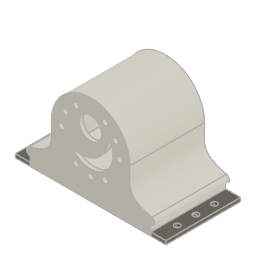
inspection_robot_01 (Autodesk Fusion 360 archive; units mm, degrees)
design "Motor Holder - JGB37-520"
Autodesk Fusion 360 part; units mm, degrees
sketch "Sketch1" plane through (0, 0, 0) normal (0, 1, 0) x (1, 0, 0)
  spline S0 degree 3 poles (32.2186, -5) (32.4791, -5) (32.737, -5.0509) (33.2189, -5.2486) (33.4382, -5.3936) (33.8089, -5.7595) (33.9568, -5.9769) (34.1608, -6.4561) (34.2151, -6.7133) (34.2219, -7.2342) (34.1744, -7.4927) (33.983, -7.9772) (33.8409, -8.1984) (33.5297, -8.5221) (33.3803, -8.6389) (33.0533, -8.8273) (32.8773, -8.8978) (32.6941, -8.9427) knots 0 0 0 0 0.078129 0.078129 0.156258 0.156258 0.234387 0.234387 0.312516 0.312516 0.390644 0.390644 0.468773 0.468773 0.525375 0.525375 0.581976 0.581976 0.581976 0.581976
  spline S1 degree 3 poles (32.6941, -8.9427) (29.0069, -9.845) (26.7125, -10.8301) (23.8662, -12.5388) (23.0225, -13.3268) (21.8903, -14.8113) (21.5152, -15.5908) (20.97, -17.528) (20.8705, -18.6908) (20.8263, -21.8742) (20.9873, -23.9601) (20.9873, -27) knots 0 0 0 0 1.138808 1.138808 2.091056 2.091056 2.992987 2.992987 4.085417 4.085417 5.724443 5.724443 5.724443 5.724443
  circle A0 centre (-0.0127, -34) radius 6
  spline S2 degree 3 poles (-32.7195, -8.9427) (-32.9724, -8.8808) (-33.2109, -8.77) (-33.6319, -8.4634) (-33.8105, -8.2705) (-34.0836, -7.8269) (-34.1756, -7.5806) (-34.2598, -7.0666) (-34.2514, -6.8039) (-34.1342, -6.2964) (-34.0266, -6.0565) (-33.7256, -5.6314) (-33.535, -5.4504) (-33.1557, -5.2099) (-32.9828, -5.1319) (-32.6205, -5.0267) (-32.4327, -5) (-32.2441, -5) knots 0 0 0 0 0.078129 0.078129 0.156258 0.156258 0.234387 0.234387 0.312516 0.312516 0.390644 0.390644 0.468773 0.468773 0.525375 0.525375 0.581976 0.581976 0.581976 0.581976
  circle A1 centre (7.7373, -13.5766) radius 1.5
  line L0 (32.2186, -5) -> (32.2186, 0)
  circle A2 centre (7.7373, -40.4234) radius 1.5
  arc A3 (9.7096, -34.034) -> (-9.7039, -19.9233) centre (-0.0127, -27) ccw
  arc A4 (-21.0127, -27) -> (20.9873, -27) centre (-0.0127, -27) ccw
  circle A5 centre (-0.0127, -11.5) radius 1.5
  spline S3 degree 3 poles (-21.0127, -27) (-21.0127, -21.6083) (-20.4943, -18.5071) (-21.8096, -15.0156) (-22.2712, -14.2366) (-23.6233, -12.8057) (-24.5151, -12.1033) (-27.7492, -10.3649) (-30.1557, -9.5701) (-32.7195, -8.9427) knots 0 0 0 0 1.617502 1.617502 2.113141 2.113141 2.569404 2.569404 3.248781 3.248781 3.248781 3.248781
  line L1 (-32.2441, 0) -> (-32.2441, -5)
  circle A6 centre (-13.4361, -34.75) radius 1.5
  circle A7 centre (-7.7627, -40.4234) radius 1.5
  circle A8 centre (13.4107, -34.75) radius 1.5
  circle A9 centre (-15.5127, -27) radius 1.5
  circle A10 centre (15.4873, -27) radius 1.5
  circle A11 centre (-7.7627, -13.5766) radius 1.5
  arc A12 (9.7096, -34.034) -> (-9.7039, -19.9233) centre (-5.2887, -34.2587) ccw
  line L2 (32.2186, 0) -> (-32.2441, 0)
  point P0 (-67.8, -16)
  constraint perpendicular L1 L2
extrude "Extrude1" add sketch "Sketch1" along normal blind 40 makes body 1
sketch "Sketch2" plane through (0, 40, 0) normal (0, 1, 0) x (-1, 0, 0)
  circle A0 centre (13.4361, 34.75) radius 1.5
  circle A1 centre (0.0127, 11.5) radius 1.5
  circle A2 centre (-15.4873, 27) radius 1.5
  circle A3 centre (-7.7373, 40.4234) radius 1.5
  circle A4 centre (7.7627, 40.4234) radius 1.5
  circle A5 centre (-13.4107, 34.75) radius 1.5
  circle A6 centre (7.7627, 13.5766) radius 1.5
  arc A7 (-9.7096, 34.034) -> (9.7039, 19.9233) centre (0.0127, 27) ccw
  arc A8 (-9.7096, 34.034) -> (9.7039, 19.9233) centre (5.2887, 34.2587) ccw
  circle A9 centre (15.5127, 27) radius 1.5
  line L0 (-32.2186, 5) -> (-32.2186, 0)
  line L1 (-32.2186, 0) -> (32.2441, 0)
  line L2 (32.2441, 0) -> (32.2441, 5)
  spline S0 degree 3 poles (32.2441, 5) (32.4327, 5) (32.6205, 5.0267) (32.9828, 5.1319) (33.1557, 5.2099) (33.535, 5.4504) (33.7256, 5.6314) (34.0266, 6.0565) (34.1342, 6.2964) (34.2514, 6.8039) (34.2598, 7.0666) (34.1756, 7.5806) (34.0836, 7.8269) (33.8105, 8.2705) (33.6319, 8.4634) (33.2109, 8.77) (32.9724, 8.8808) (32.7195, 8.9427) knots -0.581976 -0.581976 -0.581976 -0.581976 -0.525375 -0.525375 -0.468773 -0.468773 -0.390644 -0.390644 -0.312516 -0.312516 -0.234387 -0.234387 -0.156258 -0.156258 -0.078129 -0.078129 0 0 0 0
  spline S1 degree 3 poles (32.7195, 8.9427) (30.1557, 9.5701) (27.7492, 10.3649) (24.5151, 12.1033) (23.6233, 12.8057) (22.2712, 14.2366) (21.8096, 15.0156) (20.4943, 18.5071) (21.0127, 21.6083) (21.0127, 27) knots -3.248781 -3.248781 -3.248781 -3.248781 -2.569404 -2.569404 -2.113141 -2.113141 -1.617502 -1.617502 0 0 0 0
  arc A10 (21.0127, 27) -> (-20.9873, 27) centre (0.0127, 27) ccw
  spline S2 degree 3 poles (-20.9873, 27) (-20.9873, 23.9601) (-20.8263, 21.8742) (-20.8705, 18.6908) (-20.97, 17.528) (-21.5152, 15.5908) (-21.8903, 14.8113) (-23.0225, 13.3268) (-23.8662, 12.5388) (-26.7125, 10.8301) (-29.0069, 9.845) (-32.6941, 8.9427) knots -5.724443 -5.724443 -5.724443 -5.724443 -4.085417 -4.085417 -2.992987 -2.992987 -2.091056 -2.091056 -1.138808 -1.138808 0 0 0 0
  spline S3 degree 3 poles (-32.6941, 8.9427) (-32.8773, 8.8978) (-33.0533, 8.8273) (-33.3803, 8.6389) (-33.5297, 8.5221) (-33.8409, 8.1984) (-33.983, 7.9772) (-34.1744, 7.4927) (-34.2219, 7.2342) (-34.2151, 6.7133) (-34.1608, 6.4561) (-33.9568, 5.9769) (-33.8089, 5.7595) (-33.4382, 5.3936) (-33.2189, 5.2486) (-32.737, 5.0509) (-32.4791, 5) (-32.2186, 5) knots -0.581976 -0.581976 -0.581976 -0.581976 -0.525375 -0.525375 -0.468773 -0.468773 -0.390644 -0.390644 -0.312516 -0.312516 -0.234387 -0.234387 -0.156258 -0.156258 -0.078129 -0.078129 0 0 0 0
  circle A11 centre (-7.7373, 13.5766) radius 1.5
  circle A12 centre (0.0127, 34) radius 6
  arc A13 (-30.2186, 5) -> (-32.2186, 7) centre (-32.2186, 5) ccw
  line L3 (-30.2186, 5) -> (-30.2186, 2)
  line L4 (-30.2186, 2) -> (30.2441, 2)
  line L5 (30.2441, 2) -> (30.2441, 5)
  arc A14 (32.2441, 7) -> (30.2441, 5) centre (32.2441, 5) ccw
  spline S4 degree 3 poles (32.2441, 7) (30.0664, 7.5329) (27.9694, 8.1855) (26.0904, 9.0394) (25.0511, 9.5117) (24.0752, 10.0585) (23.2877, 10.6098) (21.859, 11.6099) (20.9185, 12.6606) (20.2543, 13.8079) (19.4466, 15.2031) (19.118, 16.6388) (18.9734, 18.1049) (18.7442, 20.4278) (18.9801, 22.9083) (19.0095, 26.2682) (19.0116, 26.5073) (19.0127, 26.7511) (19.0127, 27) knots -3.248781 -3.248781 -3.248781 -3.248781 -2.693258 -2.693258 -2.693258 -2.385986 -2.385986 -2.385986 -1.8285 -1.8285 -1.8285 -1.150567 -1.150567 -1.150567 -0.076448 -0.076448 -0.076448 0 0 0 0
  arc A15 (19.0127, 27) -> (-18.9873, 27) centre (0.0127, 27) ccw
  spline S5 degree 3 poles (-18.9873, 27) (-18.9873, 24.4074) (-18.8645, 22.5149) (-18.851, 20.716) (-18.8392, 19.1364) (-18.8988, 17.6011) (-19.3003, 16.0833) (-19.5893, 14.9906) (-20.0656, 13.9418) (-20.7557, 13.0031) (-21.5486, 11.9248) (-22.6816, 10.8847) (-24.3518, 9.9169) (-26.1076, 8.8994) (-28.5437, 7.8994) (-32.2186, 7) knots -5.724443 -5.724443 -5.724443 -5.724443 -4.293332 -4.293332 -4.293332 -3.036675 -3.036675 -3.036675 -2.132017 -2.132017 -2.132017 -1.092667 -1.092667 -1.092667 0 0 0 0
  dimension "d3" = -2
extrude "Extrude2" cut sketch "Sketch2" against normal up to surface (38 mm away) contours A13 L3 L4 L5 A14 S4 A15 S5 bodies 1
sketch "Sketch3" plane through (-32.2441, 0, 0) normal (-1, 0, 0) x (0, -1, 0)
  line L0 (0, 0) -> (0, 5)
  line L1 (0, 5) -> (-40, 5)
  line L2 (-40, 5) -> (-40, 0)
  line L3 (-40, 0) -> (0, 0)
  line L4 (-40, 0) -> (0, 0)
  line L5 (0, 0) -> (0, 2)
  line L6 (0, 2) -> (-40, 2)
  line L7 (-40, 2) -> (-40, 0)
  dimension "d6" = 2
  constraint horizontal L4
  constraint vertical L5
  constraint horizontal L6
  constraint vertical L7
  constraint coincident L2.end L3.start
  measures "d6" distance of L2.end L6.end
extrude "Extrude3" add sketch "Sketch3" along normal blind 8 separate body contours L0 L2 L3 L4 L5 L6 L7 makes body 2
mirror "Mirror1" about plane through (0, 0, 0) normal (1, 0, 0) of "Extrude3" makes body 3
sketch "Sketch4" plane through (0, 0, 2) normal (0, 0, 1) x (-1, 0, 0)
  line L0 (32.2441, -40) -> (40.2441, -40)
  line L1 (40.2441, -40) -> (40.2441, 0)
  line L2 (40.2441, 0) -> (32.2441, 0)
  line L3 (-40.2441, -40) -> (-40.2441, 0)
  line L4 (40.2441, -20) -> (-40.2441, -20)
  line L5 (36.2441, 0) -> (36.2441, -40)
  circle A0 centre (36.2441, -20) radius 1.5
  circle A1 centre (36.2441, -10) radius 1.5
  circle A2 centre (36.2441, -30) radius 1.5
  line L6 (-20.9873, -40) -> (21.0127, -40)
  line L7 (0, 0) -> (0.0127, -40)
  line L8 (-40.2313, -20.0256) -> (40.2568, -19.9744)
  line L9 (-32.2186, -40.0205) -> (-40.2186, -40.0256)
  circle A3 centre (-36.2377, -10.023) radius 1.5
  line L10 (-32.2441, -0.0205) -> (-32.2186, -40.0205)
  line L11 (-40.2441, -0.0256) -> (-32.2441, -0.0205)
  circle A4 centre (-36.2313, -20.023) radius 1.5
  line L12 (-40.2186, -40.0256) -> (-40.2441, -0.0256)
  line L13 (-36.2441, -0.023) -> (-36.2186, -40.023)
  circle A5 centre (-36.225, -30.023) radius 1.5
  line L14 (32.2441, 0) -> (32.2441, -40)
  point P0 (36.2441, -20)
  point P1 (-36.2313, -20.023)
  dimension "d11" = 3
  dimension "d14" = 10
  dimension "d15" = 0
  constraint midpoint L1 L4.start
  constraint midpoint L3 L4.end
  constraint midpoint L2 L5.start
  constraint midpoint L0 L5.end
  constraint midpoint L5 P0
  constraint coincident L5 P0
  constraint coincident P0 A0.centre
  constraint coincident L7.start origin
  constraint midpoint L6 L7.end
  constraint symmetric L2.end L7 L10.start
  constraint symmetric L0.start L7 L9.start
  constraint symmetric L0.end L7 L9.end
  constraint symmetric L1.end L7 L11.start
  constraint symmetric L4.start L7 L8.start
  constraint symmetric L4.end L7 L8.end
  constraint symmetric L5.start L7 L13.start
  constraint symmetric L5.end L7 L13.end
  constraint symmetric P0 L7 P1
  constraint symmetric A0 L7 A4
  constraint symmetric A1 L7 A3
  constraint symmetric A2 L7 A5
  measures "d11" diameter of A0
extrude "Extrude4" cut sketch "Sketch4" against normal through all contours L5 A2 | L5 A2 | L4 L5 A0 L8 | L4 L5 A0 | L4 L5 A0 L8 | L4 L5 A0 | L5 A0 L8 | L5 A0 L8 | L4 A4 L13 | L8 A4 L13 | L5 A1 | L5 A1 | L4 A4 L13 | L8 A4 L13 | A3 L13 | A3 L13 | L13 A5 | L13 A5 bodies 2 1 3
sketch "Sketch5" plane through (0, 0, 2) normal (0, 0, 1) x (-1, 0, 0)
  line L0 (30.2441, -2) -> (-30.2186, -2)
  line L1 (-30.2186, -2) -> (-30.2186, -40)
  line L2 (-30.2186, -40) -> (30.2441, -40)
  line L3 (30.2441, -40) -> (30.2441, -2)
  line L4 (0.0127, -2) -> (0.0127, -40) construction
  line L5 (0.0127, -21) -> (-30.2186, -21) construction
  line L6 (-15.103, -21) -> (-15.103, -2) construction
  circle A0 centre (-15.103, -11.5) radius 1.5
  circle A1 centre (-15.103, -30.5) radius 1.5
  circle A2 centre (15.1284, -11.5) radius 1.5
  circle A3 centre (15.1284, -30.5) radius 1.5
  point P0 (-15.103, -11.5)
  dimension "d17" = 3
  constraint midpoint L0 L4.start
  constraint midpoint L2 L4.end
  constraint midpoint L4 L5.start
  constraint midpoint L1 L5.end
  constraint midpoint L5 L6.start
  constraint coincident L0 L6.end
  constraint perpendicular L0 L6
  constraint midpoint L6 P0
  constraint coincident P0 A0.centre
  constraint symmetric L5 A0 A1
  constraint symmetric L4 A0 A2
  constraint symmetric L4 A1 A3
  measures "d17" diameter of A0
extrude "Extrude5" cut sketch "Sketch5" against normal through all contours A0 | A1 | A2 | A3 bodies 2 1
